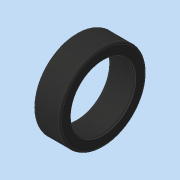
# Autodesk Inventor part: 橡胶外轮设计
Saved by Autodesk Inventor 2019 (Build 230136000, 136)
## iProperties
Created: 2020-10-29
Part Number: 橡胶外轮设计
Material: 橡胶
Document SubType Name: Modeling
Designer: Wang Hua
Density: 0.93 g/cm^3
Appearance: 橡胶 - 黑色
Author: Wang Hua
Autodesk Inventor part; units mm, degrees
ref_plane "YZ Plane" through (0, 0, 0) normal (1, 0, 0) x (0, 1, 0)
ref_plane "XZ Plane" through (0, 0, 0) normal (0, 1, 0) x (-1, 0, 0)
ref_plane "XY Plane" through (0, 0, 0) normal (0, 0, 1) x (1, 0, 0)
sketch "草图1" plane through (0, 0, 0) normal (0, 0, 1) x (1, 0, 0)
  line L0 (-7.5, 24.5) -> (7.5, 24.5)
  line L1 (-10.9677, 0) -> (10.5779, 0) projected
  line L2 (0, -103.0462) -> (0, 45.7577) projected
  line L3 (-7.5, 24.5) -> (-7.5, 18.5)
  line L4 (-7.5, 18.5) -> (-7, 18.5)
  arc A0 (-6.5, 18) -> (-7, 18.5) centre (-7, 18) ccw
  line L5 (-7, 18) -> (-7.8897, 18) construction
  line L6 (7.5, 24.5) -> (7.5, 18.5)
  line L7 (7.5, 18.5) -> (7, 18.5)
  arc A1 (7, 18.5) -> (6.5, 18) centre (7, 18) ccw
  arc A2 (6.5, 18) -> (-6.5, 18) centre (0, -81.7885) ccw
  point P0 (0, 0)
  dimension "d1" = 0.5
  dimension "d2" = 6
  dimension "d3" = 1
  dimension "d4" = 24.5
  dimension "d11" = 15
  dimension "d13" = 100
  dimension "d14" = 18
  constraints: 12 end point, 6 point on circle, 5 symmetric about line, 3 centre point, 2 horizontal, 1 parallel, 1 point on line, 1 vertical, 1 other
  measures "d1" distance of L3.end L4.end
  measures "d2" distance of L0.start L3.end
  measures "d3" diameter of A0
  measures "d4" distance between parallel lines of L1 L0
  measures "d11" distance of L0.start L0.end
  measures "d13" radius of A2
  measures "d14" distance from line of L1 A1.end
revolve "旋转1" add sketch "草图1" angle 360 about axis through (-10, 0, 0) along (1, 0, 0)
fillet "圆角1" radius 1 2 edges at (-7.5, -24.5, 0) (7.5, -24.5, 0)
